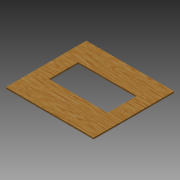
# Autodesk Inventor part: drzwiczki-przod
Saved by Autodesk Inventor 2013 (Build 170138000, 138)
## iProperties
Created: 2014-04-26
Part Number: drzwiczki-przod
Material: Generic
Document SubType Name: Modeling
Designer: Masta
Density: 1 g/cm^3
Author: Masta
Autodesk Inventor part; units mm, degrees
ref_plane "YZ Plane" through (0, 0, 0) normal (1, 0, 0) x (0, 1, 0)
ref_plane "XZ Plane" through (0, 0, 0) normal (0, 1, 0) x (-1, 0, 0)
ref_plane "XY Plane" through (0, 0, 0) normal (0, 0, 1) x (1, 0, 0)
sketch "Sketch1" plane through (0, 0, 0) normal (0, 0, 1) x (1, 0, 0)
  line L0 (-300, -275) -> (300, -275)
  line L1 (300, -275) -> (300, 275)
  line L2 (300, 275) -> (-300, 275)
  line L3 (-300, 275) -> (-300, -275)
  line L4 (-300, -275) -> (300, 275) construction
  line L5 (300, -275) -> (-300, 275) construction
  line L6 (-200, -80) -> (200, -80)
  line L7 (200, -80) -> (200, 120)
  line L8 (200, 120) -> (-200, 120)
  line L9 (-200, 120) -> (-200, -80)
  line L10 (-200, -80) -> (200, 120) construction
  line L11 (200, -80) -> (-200, 120) construction
  line L12 (0, 20) -> (0, 0) construction
  dimension "d0" = 600
  dimension "d1" = 550
  dimension "d4" = 400
  dimension "d5" = 200
  dimension "d6" = 20
  constraints: 26 end point, 5 parallel, 4 midpoint, 2 horizontal, 2 perpendicular
  measures "d0" distance of L2.end L1.end
  measures "d1" distance of L1.end L0.end
  measures "d4" distance of L8.end L7.end
  measures "d5" distance of L7.end L6.end
  measures "d6" distance of L12.start L12.end
extrude "Extrusion1" add sketch "Sketch1" along normal blind 10
body "Solid1"
